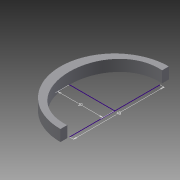
# Autodesk Inventor part: BassGuitarCurveTest
Saved by Autodesk Inventor 2015 (Build 190159000, 159)
## iProperties
Created: 2016-04-08
Part Number: BassGuitarCurveTest
Material: Generic
Document SubType Name: Modeling
Designer: Hatch
Density: 1 g/cm^3
Appearance: Default
Author: Hatch
Autodesk Inventor part; units mm, degrees
ref_plane "YZ Plane" through (0, 0, 0) normal (1, 0, 0) x (0, 1, 0)
ref_plane "XZ Plane" through (0, 0, 0) normal (0, 1, 0) x (-1, 0, 0)
ref_plane "XY Plane" through (0, 0, 0) normal (0, 0, 1) x (1, 0, 0)
sketch "Sketch1" plane through (0, 0, 0) normal (0, 1, 0) x (-1, 0, 0)
  line L0 (0, 0) -> (0, -40)
  line L1 (0, -20) -> (20, -20)
  dimension "d0" = 40
  dimension "d1" = 20
  constraints: 4 end point, 1 horizontal, 1 midpoint, 1 vertical
  measures "d0" distance of L0.start L0.end
  measures "d1" distance of L1.start L1.end
sketch "Sketch2" plane through (0, 0, 0) normal (0, 1, 0) x (-1, 0, 0)
  arc A0 (0, -40) -> (0, 0) centre (0, -20) ccw
  line L0 (0, 0) -> (0, 1)
  line L1 (0, -40) -> (0, -41)
  line L2 (0, -20) -> (14.8492, -5.1508) construction
  line L3 (0, -20) -> (0, 1) construction
  spline S0 degree 4 poles (0, 1) (18.89, 2.2775) (28.1468, -20.0014) (18.8898, -42.2749) (0, -41) knots 0 0 0 0 0 1 1 1 1 1
  line L4 (0, 1) -> (0, 4)
  line L5 (0, 4) -> (5, 4)
  line L6 (0, -41) -> (0, -44)
  line L7 (0, -44) -> (5, -44)
  line L8 (20, -20) -> (23, -20)
  arc A1 (24, -20) -> (0, 4) centre (0, -20) ccw
  arc A2 (0, -44) -> (24, -20) centre (0, -20) ccw
  point P0 (14.8493, -34.8486)
  dimension "d4" = 1
  dimension "d5" = 1
  dimension "d6" = 45
  dimension "d7" = 3
  dimension "d8" = 5
  dimension "d9" = 3
  dimension "d10" = 5
  dimension "d11" = 3
  constraints: 18 end point, 7 point on circle, 4 vertical, 3 centre point, 2 coincident, 2 perpendicular, 1 horizontal, 5 other
  measures "d4" distance of L0.start L0.end
  measures "d5" distance of L1.start L1.end
  measures "d6" angle of L2 L3
  measures "d7" distance of L0.end L4.end
  measures "d8" distance of L4.end L5.end
  measures "d9" distance of L1.end L6.end
  measures "d10" distance of L6.end L7.end
  measures "d11" distance of L8.start L8.end
extrude "Extrusion1" add sketch "Sketch2" along normal blind 5 contours S0 L4 A1 A2 L6
body "Solid1"
